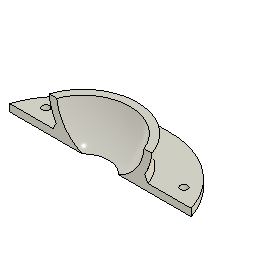
SupportTennisBall v5 (Autodesk Fusion 360 design; units mm, degrees)
Autodesk Fusion 360 part; units mm, degrees
note: some values were not read from the file. Set by a fixed rule: which face or edge a step refers to.
sketch "Sketch1" plane through (0, 0, 0) normal (1, 0, 0) x (0, 1, 0)
  line L0 (0, 0) -> (58.0426, 0)
  line L1 (58.0426, 0) -> (58.0426, 29.3578)
  line L2 (58.0426, 29.3578) -> (0, 29.3578)
  line L3 (0, 29.3578) -> (0, 0)
  dimension "d18" = 29.3578
  constraint horizontal L0
  constraint vertical L1
  constraint horizontal L2
  constraint vertical L3
  constraint coincident L0.start L3.end
  measures "d18" distance of L0.end L1.end
sketch "Sketch1 (2)" plane through (0, 0, 0) normal (1, 0, 0) x (0, 1, 0) in component "ball"
  circle A0 centre (0, 32.5) radius 32.5
  line L0 (0, 65) -> (0, 0)
  dimension "d1" = 65
  dimension "d2" = 32.5
  constraint vertical L0.end A0.centre
  constraint coincident A0 L0.start
  constraint coincident A0 L0.end
  constraint vertical L0
  constraint vertical A0.centre L0.end
  measures "d1" diameter of A0
  measures "d2" vertical distance of L0.end A0.centre
revolve "Revolve1" add sketch "Sketch1 (2)" angle 360 about axis through (0, 0, 65) along (0, 0, -1) contours A0 L0 picked at (20.8695, 31.8345) makes body 1 in component "ball"
ref_plane "WorkPlane1" through (0, 12, 0) normal (0, 1, 0) x (0, 0, 1)
extrude "Extrude1" add sketch "Sketch1" along normal mid plane 180 separate body makes body 2
copy_body "CopyPasteBodies1" bodies 1 makes body 3
combine "Combine1" operation cut target body 2 tool bodies 3 keep tools
shell "Shell1" thickness 10 outward yes removed faces 0 bodies 3
combine "Combine2" operation intersect target body 2 tool bodies 3
sketch "Sketch2" plane through (0, 0, 0) normal (0, 0, 1) x (1, 0, 0)
  line L0 (-65, 0) -> (65, 0)
  line L1 (65, 0) -> (65, 50)
  line L2 (65, 50) -> (-65, 50)
  line L3 (-65, 50) -> (-65, 0)
  arc A0 (42.3837, 0) -> (-42.3837, 0) centre (0, 0) ccw construction
  arc A1 (52.3837, 0) -> (-52.3837, 0) centre (0, 0) ccw construction
  circle A2 centre (-47.54, 22) radius 2.5
  line L4 (65, 12) -> (-65, 12) construction
  circle A3 centre (47.54, 22) radius 2.5
  point P0 (-47.54, 22)
  dimension "d7" = 10
  dimension "d8" = 5
  dimension "d15" = 130
  dimension "d16" = 50
  dimension "d22" = 12
  dimension "d26" = 5
  dimension "d27" = 10
  constraint horizontal L0
  constraint vertical L1
  constraint horizontal L2
  constraint vertical L3
  constraint midpoint A0.centre L0
  constraint coincident P0 A2.centre
  constraint coincident P0 A1
  constraint coincident L1 L4.start
  constraint coincident L3 L4.end
  constraint perpendicular L3 L4
  constraint coincident A1 A3.centre
  constraint horizontal P0 A3.centre
  measures "d8" diameter of A2
  measures "d15" distance of L1.end L2.end
  measures "d16" distance of L0.start L2.end
  measures "d22" distance of L0 L4
  measures "d26" diameter of A3
  measures "d27" distance of L4 A3.centre
extrude "Extrude2" add sketch "Sketch2" along normal blind 10 bodies 2
delete_face "DeleteFace1" 1 faces at (4.874, 6.1119, 10) on bodies 2
fillet "Fillet1" radius 55 2 edges at (-65, 50, 5) (65, 50, 5) on bodies 2
split "Split1" by plane through (0, 12, 0) normal (0, 1, 0) bodies 2 makes body 4 at (-3.4092, 30.6102, 0)
move_face "OffsetFaces1" offset -5 1 faces at (-3.4092, 30.6102, 0) on bodies 4
move_face "OffsetFaces2" offset -5 1 faces at (0, 41.8016, 24.827) on bodies 4
chamfer "Chamfer2" distance 5 angle 45 1 edges at (0, 30, 10) on bodies 4
component "ball" placed x (1, 0, 0) y (0, 1, 0) z (0, 0, 1) at (0, 0, 0)
hidden bodies 2
equation "d2 = d1 / 2"
equation "d26 = d8"
